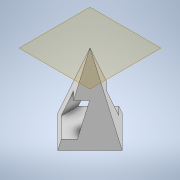
# Autodesk Inventor part: Деталь2
Saved by Autodesk Inventor 2021.2 (Build 252289000, 289)
## iProperties
Created: 2023-10-05
Part Number: Деталь2
Material: Типовые
Document SubType Name: Modeling
Designer: User
Density: 1 g/cm^3
Appearance: По умолчанию
Author: User
Autodesk Inventor part; units mm, degrees
ref_plane "YZ Plane" through (0, 0, 0) normal (1, 0, 0) x (0, 1, 0)
ref_plane "XY Plane" through (0, 0, 0) normal (0, 0, 1) x (1, 0, 0)
sketch "Эскиз1" plane through (0, 0, 0) normal (0, 1, 0) x (-1, 0, 0)
  circle A0 centre (0, 0) radius 40
  line L0 (40, 0) -> (0, -40)
  line L1 (0, -40) -> (-40, 0)
  line L2 (-40, 0) -> (0, 40)
  line L3 (0, 40) -> (40, 0)
  dimension "d0" = 80
  constraints: 8 end point, 2 coincident, 1 horizontal alignment, 11 other
ref_plane "РабПлоскость1" through (0, 90, 0) normal (0, 1, 0) x (-1, 0, 0)
sketch "Эскиз2" plane through (0, 90, 0) normal (0, 1, 0) x (-1, 0, 0)
  point P0 (0, 0)
  point P1 (0, 0)
  constraints: 1 coincident
loft "Лофт1" add profiles "Эскиз1" section 1 point at (0, 90, 0) contours L0 L1 L2 L3
sketch "Эскиз3" plane through (0, 0, 0) normal (0, 0, 1) x (1, 0, 0)
  line L0 (0, 0) -> (0, 10)
  line L1 (0, 90) -> (0, 0) projected
  line L2 (0, 10) -> (10, 10)
  line L3 (10, 10) -> (10, 44)
  line L4 (10, 44) -> (-10, 44)
  line L5 (0, 10) -> (-25, 10)
  line L6 (-25, 10) -> (-10, 44)
  constraints: 12 end point, 3 perpendicular, 1 horizontal, 1 point on line
extrude "Выдавливание1" cut sketch "Эскиз3" against normal mid plane 90
